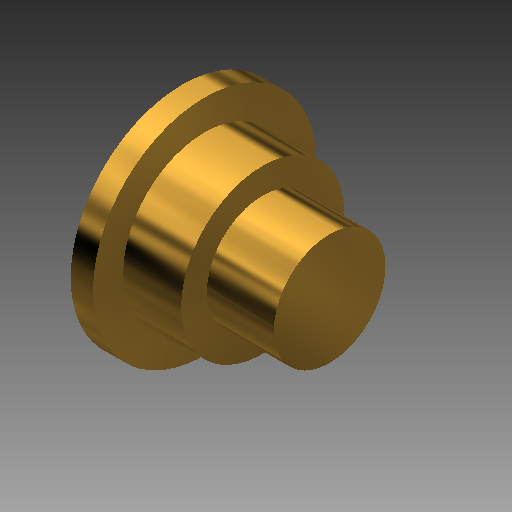
# Autodesk Inventor part: 403-09
Saved by Autodesk Inventor 2019 (Build 230136000, 136)
## iProperties
Company: Autodesk Inc.
Created: 2017-06-27
Part Number: 403-09
Material: Brass, Soft Yellow
Document SubType Name: Modeling
Designer: Autodesk Inc.
Mass: 0.260733 g
Surface Area: 0.738117 cm^2
Volume: 0.0307831 cm^3
Density: 8.47 g/cm^3
Appearance: Brass - Satin
Author: Inventor
Autodesk Inventor part; units mm, degrees
ref_plane "YZ Plane" through (0, 0, 0) normal (1, 0, 0) x (0, 1, 0)
ref_plane "XZ Plane" through (0, 0, 0) normal (0, 1, 0) x (-1, 0, 0)
ref_plane "XY Plane" through (0, 0, 0) normal (0, 0, 1) x (1, 0, 0)
sketch "Sketch1" plane through (0, 0, 0) normal (0, 0, 1) x (1, 0, 0)
  line L0 (0, 0) -> (0.5, 0)
  line L1 (0.5, 0) -> (0.5, 2.5)
  line L2 (0.5, 2.5) -> (0, 2.5)
  line L3 (0, 2.5) -> (0, 0)
  line L4 (0.5, 0) -> (1.8, 0)
  line L5 (1.8, 0) -> (1.8, 1.825)
  line L6 (1.8, 1.825) -> (0.5, 1.825)
  line L7 (0.5, 1.825) -> (0.5, 0)
  line L8 (1.8, 0) -> (3.3, 0)
  line L9 (3.3, 0) -> (3.3, 1.25)
  line L10 (3.3, 1.25) -> (1.8, 1.25)
  line L11 (1.8, 1.25) -> (1.8, 0)
  dimension "d0" = 0.5
  dimension "d1" = 1.8
  dimension "d2" = 3.3
  dimension "d3" = 2.5
  dimension "d4" = 3.65
  dimension "d5" = 5
  constraints: 24 end point, 6 parallel, 3 horizontal, 3 perpendicular
  measures "d0" distance of L1.end L2.end
  measures "d1" distance between parallel lines of L5 L3
  measures "d2" distance between parallel lines of L9 L3
  measures "d3" diameter of L10 L8
  measures "d4" diameter of L6 L8
  measures "d5" diameter of L2 L8
revolve "Revolution1" add sketch "Sketch1" angle 360 about axis through (1.8, 0, 0) along (1, 0, 0)
body "Solid1"
